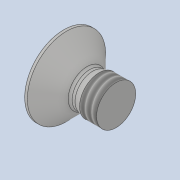
# Autodesk Inventor part: SFBJ6-8
Saved by Autodesk Inventor 2022 (Build 260153000, 153)
## iProperties
Category: PARTsolutions
Company: MISUMI
Created: 2023-06-20
Part Number: SFBJ6-8
Material: Generic
Catalog Web Link: www.cadenas.de
Description: BFBJ, SFBJ-Cross Recessed Flat Head Machine Screws
Vendor: MISUMI
Document SubType Name: Modeling
Designer: psAdmin
Manufacturer: MISUMI
Mass: 0.331704 g
Surface Area: 4.05278 cm^2
Volume: 0.331704 cm^3
Density: 1 g/cm^3
Appearance: PSOLRGB-175-175-175
PSOL_IDENT_0: {$CADENAS_DATA/23d-libs/misumi/metric/27_screws_nuts/sfbj.prj},164 {VTYP=3D},{NB=SFBJ6-8},{LINA=SFBJ
PSOL_IDENT_1: 6-8},{NN=BFBJ, SFBJ},{DATE=29.05.2023 07:55:08},{GEOMDATE=15.12.2011 00:00:00},{VERSION=},{LINEID=60
PSOL_IDENT_2: },{WBVAR=MAT,L},{WBNUMERIC=L}  {NB=SFBJ6-8},{LINA=SFBJ6-8},{KT=DUMMY},{PN=SFBJ6-8},{TYPE=SFBJ},{MAT=
PSOL_IDENT_3: SUS304},{MATA='SWCH','SWCH Carbon Steel','SUS304','304 Stainless Steel'},{M=6},{M1=6.0},{L=8},{LA=8,
PSOL_IDENT_4: 10,12,15,20},{P=1.00},{MP=6x1.0},{A=12.0},{E=3.40},{MM=6.700},{CC=0.400},{RR=0.600}
NB: SFBJ6-8
NN: BFBJ, SFBJ
NT: Cross Recessed Flat Head Machine Screws
NBSYN: $PN.
LINA: SFBJ6-8
CATALOG: Misumi
PN: SFBJ6-8
MAT: 304 Stainles Steel Equivalent
M: 6
L: 8
MP: 6x1.0
A: 12
E: 3.4
SUPPLIER: MISUMI
ARTICLENO: SFBJ6-8
BOMINFO: SFBJ6-8
CREATOR: CADENAS GmbH
Title: SFBJ6-8
Author: Cadenas PARTsolutions
Comments: Cross Recessed Flat Head Machine Screws
Autodesk Inventor part; units mm, degrees
sketch "Sketch_1" plane through (0, 0, 0) normal (0, 0, 1) x (1, 0, 0)
  line L0 (4.6, 0) -> (-3.4, 0)
  line L1 (-3.4, 0) -> (-3.4, 6)
  line L2 (-3.4, 6) -> (-3, 6)
  line L3 (-3, 6) -> (0.131, 2.869)
  arc A0 (0.131, 2.869) -> (0.5553, 2.6932) centre (0.5553, 3.2932) ccw
  line L4 (0.5553, 2.6932) -> (1, 2.6932)
  line L5 (1, 2.6932) -> (2, 3)
  line L6 (2, 3) -> (4.6, 3)
  line L7 (4.6, 3) -> (4.6, 0)
  line L8 (4.6, 0) -> (-3.4, 0)
  constraints: 18 end point, 2 point on circle, 1 centre point
revolve "Revolution1" add sketch "Sketch_1" angle 360 about axis through (4.6, 0, 0) along (1, 0, 0)
thread "Thread1" size "M6x1" class "6g" standard "ISO Metric profile" full length
sketch "Sketch_2" plane through (-3.4, 0, 0) normal (1, 0, 0) x (0, 0, -1)
  line L0 (-3.35, -0.8) -> (-2, -0.8)
  arc A0 (-0.8, -2) -> (-2, -0.8) centre (-2, -2) ccw
  line L1 (-0.8, -2) -> (-0.8, -3.35)
  line L2 (-0.8, -3.35) -> (0.8, -3.35)
  line L3 (0.8, -3.35) -> (0.8, -2)
  arc A1 (2, -0.8) -> (0.8, -2) centre (2, -2) ccw
  line L4 (2, -0.8) -> (3.35, -0.8)
  line L5 (3.35, -0.8) -> (3.35, 0.8)
  line L6 (3.35, 0.8) -> (2, 0.8)
  arc A2 (0.8, 2) -> (2, 0.8) centre (2, 2) ccw
  line L7 (0.8, 2) -> (0.8, 3.35)
  line L8 (0.8, 3.35) -> (-0.8, 3.35)
  line L9 (-0.8, 3.35) -> (-0.8, 2)
  arc A3 (-2, 0.8) -> (-0.8, 2) centre (-2, 2) ccw
  line L10 (-2, 0.8) -> (-3.35, 0.8)
  line L11 (-3.35, 0.8) -> (-3.35, -0.8)
  constraints: 24 end point, 8 point on circle, 4 centre point
extrude "Extrusion1" cut sketch "Sketch_2" along normal blind 1.7
ref_plane "bolt_XY" through (-3.4, 0, 0) normal (1, 0, 0) x (0, 0, -1)
ref_plane "bolt_YZ" through (-3.4, 0, 0) normal (0, 0, -1) x (0, 1, 0)
ref_plane "bolt_ZX" through (-3.4, 0, 0) normal (0, 1, 0) x (1, 0, 0)
ref_plane "nut_XY" through (4.6, 0, 0) normal (1, 0, 0) x (0, 0, -1)
ref_plane "nut_YZ" through (4.6, 0, 0) normal (0, 0, -1) x (0, 1, 0)
ref_plane "nut_ZX" through (4.6, 0, 0) normal (0, 1, 0) x (1, 0, 0)
body "Solid1"
